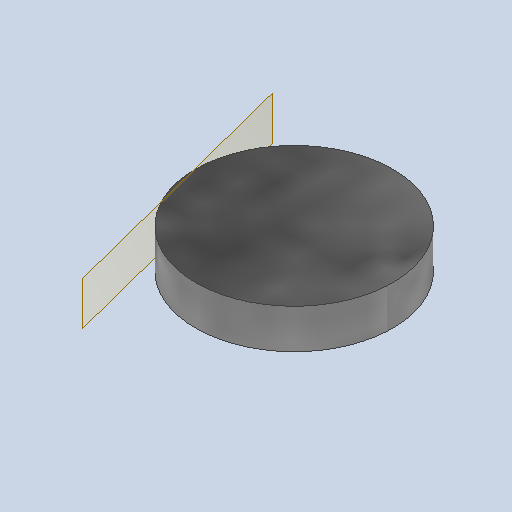
# Autodesk Inventor part: mini vibrator
Saved by Autodesk Inventor 2025.2 (Build 292293000, 293)
## iProperties
Created: 2024-12-23
Part Number: mini vibrator
Material: 一般
Document SubType Name: Modeling
Designer: naka6
Density: 1 g/cm^3
Appearance: 鋼材 メッキ
Author: naka6
Autodesk Inventor part; units mm, degrees
ref_plane "YZ Plane" through (0, 0, 0) normal (1, 0, 0) x (0, 1, 0)
ref_plane "XZ Plane" through (0, 0, 0) normal (0, 1, 0) x (-1, 0, 0)
ref_plane "XY Plane" through (0, 0, 0) normal (0, 0, 1) x (1, 0, 0)
sketch "スケッチ1" plane through (0, 0, 0) normal (0, 1, 0) x (-1, 0, 0)
  circle A0 centre (0, 0) radius 5
  dimension "d0" = 10
  constraints: 1 centre point, 1 coincident
  measures "d0" diameter of A0
extrude "押し出し1" add sketch "スケッチ1" along normal blind 2
ref_plane "作業平面1" through (-5.1207, 2.166, -0.6427) normal (0.9685804, 0, -0.2487008) x (0, -1, 0)
sketch "スケッチ2" plane through (-5.1207, 2.166, -0.6427) normal (0.9685804, 0, -0.2487008) x (0, -1, 0)
  line L0 (0.166, 3.104) -> (0.166, -6.896) projected
  line L1 (2.166, 3.104) -> (2.166, -6.896) projected
  line L2 (2.166, -6.896) -> (0.166, -6.896) projected
  line L3 (2.166, 3.104) -> (0.166, 3.104) projected
  circle A0 centre (1.166, -0.896) radius 0.25
  circle A1 centre (1.166, -2.896) radius 0.25
  point P0 (2.166, -1.896)
  dimension "d3" = 2
  dimension "d4" = 1
  dimension "d5" = 4
  dimension "d6" = 1
  dimension "d7" = 0.5
  dimension "d8" = 0.5
  constraints: 2 centre point, 2 coincident
  measures "d3" distance of point (1.166, -0.896) point (1.166, -2.896)
  measures "d4" distance from line of L1 point (1.166, -2.896)
  measures "d5" distance from line of L2 point (1.166, -2.896)
  measures "d6" distance from line of L1 point (1.166, -0.896)
  measures "d7" diameter of A0
  measures "d8" diameter of A1
extrude "押し出し2" cut sketch "スケッチ2" against normal blind 2 contours A0 | A1
